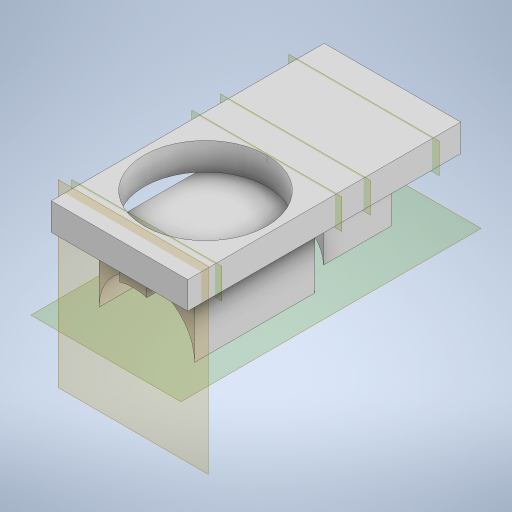
# Autodesk Inventor part: dcmotor_housing_lid
Saved by Autodesk Inventor 2023 (Build 270158000, 158)
## iProperties
Created: 2023-03-20
Part Number: dcmotor_housing_lid
Material: Generic
Document SubType Name: Modeling
Designer: caleb
Density: 1 g/cm^3
Appearance: Default
Author: caleb
Autodesk Inventor part; units mm, degrees
ref_plane "YZ Plane" through (0, 0, 0) normal (1, 0, 0) x (0, 1, 0)
ref_plane "XZ Plane" through (0, 0, 0) normal (0, 1, 0) x (-1, 0, 0)
ref_plane "XY Plane" through (0, 0, 0) normal (0, 0, 1) x (1, 0, 0)
sketch "Sketch1" plane through (0, 0, 0) normal (0, 1, 0) x (-1, 0, 0)
  line L0 (0, 0) -> (50, 0)
  line L1 (50, 0) -> (50, -100)
  line L2 (50, -100) -> (0, -100)
  line L3 (0, -100) -> (0, 0)
  line L4 (25, 0) -> (25, -100)
  line L5 (7.5, -54) -> (7.5, -10)
  line L6 (7.5, -10) -> (42.5, -10)
  line L7 (42.5, -10) -> (42.5, -54)
  line L8 (42.5, -54) -> (7.5, -54)
  line L9 (7.5, -54) -> (42.5, -10) construction
  line L10 (7.5, -10) -> (42.5, -54) construction
  line L11 (7.5, -54) -> (51.5, -54) construction
  line L12 (14.75, -64.45) -> (14.75, -89.55)
  line L13 (14.75, -89.55) -> (35.25, -89.55)
  line L14 (35.25, -89.55) -> (35.25, -64.45)
  line L15 (35.25, -64.45) -> (14.75, -64.45)
  line L16 (14.75, -64.45) -> (35.25, -89.55) construction
  line L17 (14.75, -89.55) -> (35.25, -64.45) construction
  line L18 (14.75, -64.45) -> (39.85, -64.45) construction
  line L19 (25, -10) -> (25, -15)
  line L20 (25, -10) -> (30, -10) construction
  line L21 (20, -20) -> (30, -20)
  line L22 (30, -20) -> (30, -10)
  line L23 (30, -10) -> (20, -10)
  line L24 (20, -10) -> (20, -20)
  line L25 (20, -20) -> (30, -10) construction
  line L26 (30, -20) -> (20, -10) construction
  line L27 (20, -20) -> (30, -20) construction
  line L28 (30, -15) -> (20, -15)
  line L29 (20, -10) -> (30, -10)
  line L30 (30, -10) -> (30, -5)
  line L31 (30, -5) -> (20, -5)
  line L32 (20, -5) -> (20, -10)
  line L33 (25, -54) -> (25, -64.45)
  line L34 (30, -54) -> (30, -64.45)
  line L35 (30, -64.45) -> (20, -64.45)
  line L36 (20, -64.45) -> (20, -54)
  line L37 (20, -54) -> (30, -54)
  line L38 (30, -54) -> (20, -64.45) construction
  line L39 (30, -64.45) -> (20, -54) construction
  circle A0 centre (25, -31.5) radius 22.5
  point P0 (25, -32)
  point P1 (25, -77)
  point P2 (25, -77)
  point P3 (25, -59.225)
  dimension "d36" = 45
  dimension "d0" = 50
  dimension "d1" = 100
  dimension "d2" = 44
  dimension "d3" = 90
  dimension "d4" = 35
  dimension "d5" = 10
  dimension "d6" = 25.1
  dimension "d7" = 90
  dimension "d8" = 20.5
  dimension "d9" = 5
  dimension "d10" = 90
  dimension "d11" = 0
  dimension "d23" = 10
  dimension "d24" = 5
  dimension "d25" = 10
  constraints: 80 end point, 14 midpoint, 14 parallel, 6 horizontal, 6 perpendicular, 5 point on line, 4 equal length, 1 coincident, 1 collinear, 1 vertical, 1 vertical alignment, 2 other
  measures "d0" distance of L1.end L3.start
  measures "d1" distance of L0.end L1.end
  measures "d2" distance of L5.start L6.start
  measures "d3" angle of L11 L5
  measures "d4" distance of L6.start L6.end
  measures "d5" distance between parallel lines of L6 L0
  measures "d6" distance of L15.end L17.start
  measures "d7" angle of L12 L18
  measures "d8" distance of L14.start L17.start
  measures "d9" distance of L19.start L19.end
  measures "d10" angle of L19 L20
  measures "d11" distance between parallel lines of L21 L27
  measures "d23" distance of L31.end L30.end
  measures "d24" distance of L30.end L29.end
  measures "d25" distance of L34.end L35.end
extrude "Extrusion1" add sketch "Sketch1" along normal blind 10
ref_plane "Work Plane1" through (-14.75, 0, -89.55) normal (0, 0, -1) x (-1, 0, 0)
ref_plane "Work Plane2" through (-14.75, 0, -64.45) normal (0, 0, -1) x (-1, 0, 0)
ref_plane "Work Plane3" through (-7.5, 0, -54) normal (0, 0, -1) x (-1, 0, 0)
ref_plane "Work Plane4" through (-7.5, 0, -10) normal (0, 0, -1) x (-1, 0, 0)
sketch "Sketch2" plane through (-14.75, 0, -89.55) normal (0, 0, -1) x (-1, 0, 0)
  line L0 (-14.75, 0) -> (35.25, 0) projected
  line L1 (35.25, 0) -> (35.25, 10) projected
  line L2 (-14.75, 10) -> (35.25, 10) projected
  line L3 (-14.75, 0) -> (-14.75, 10) projected
  line L4 (-14.75, 0) -> (35.25, 0)
  line L5 (35.25, 0) -> (35.25, -50)
  line L6 (35.25, -50) -> (-14.75, -50)
  line L7 (-14.75, -50) -> (-14.75, 0)
  line L8 (0, 0) -> (20.5, 0) projected
  circle A0 centre (10.25, -25) radius 10.25
  dimension "d14" = 50
  dimension "d15" = 50
  dimension "d16" = 20.5
  constraints: 8 end point, 2 parallel, 1 centre point, 1 coincident, 1 horizontal, 1 perpendicular
  measures "d14" distance of L5.end L6.end
  measures "d15" distance of L4.end L5.end
  measures "d16" diameter of A0
sketch "Sketch3" plane through (-7.5, 0, -54) normal (0, 0, -1) x (-1, 0, 0)
  line L0 (42.5, 0) -> (-7.5, 0) projected
  line L1 (-7.5, 0) -> (-7.5, 10) projected
  line L2 (42.5, 10) -> (-7.5, 10) projected
  line L3 (42.5, 0) -> (42.5, 10) projected
  line L4 (-7.5, 0) -> (42.5, 0)
  line L5 (42.5, 0) -> (42.5, -50)
  line L6 (42.5, -50) -> (-7.5, -50)
  line L7 (-7.5, -50) -> (-7.5, 0)
  line L8 (0, 0) -> (35, 0) projected
  circle A0 centre (17.5, -25) radius 17.5
  dimension "d17" = 50
  dimension "d18" = 50
  dimension "d19" = 35
  constraints: 8 end point, 2 parallel, 1 centre point, 1 coincident, 1 horizontal, 1 perpendicular
  measures "d17" distance of L5.end L6.end
  measures "d18" distance of L4.end L5.end
  measures "d19" diameter of A0
sketch "Sketch4" plane through (-14.75, 0, -64.45) normal (0, 0, -1) x (-1, 0, 0)
  line L0 (35.25, 0) -> (-14.75, 0) projected
  line L1 (-14.75, 0) -> (-14.75, 10) projected
  line L2 (35.25, 10) -> (-14.75, 10) projected
  line L3 (35.25, 0) -> (35.25, 10) projected
  line L4 (-14.75, 0) -> (35.25, 0)
  line L5 (35.25, 0) -> (35.25, -50)
  line L6 (35.25, -50) -> (-14.75, -50)
  line L7 (-14.75, -50) -> (-14.75, 0)
  circle A0 centre (10.25, -25) radius 5
  dimension "d20" = 50
  dimension "d21" = 50
  dimension "d22" = 10
  constraints: 8 end point, 2 parallel, 1 centre point, 1 coincident, 1 horizontal, 1 perpendicular
  measures "d20" distance of L5.end L6.end
  measures "d21" distance of L4.end L5.end
  measures "d22" diameter of A0
ref_plane "Work Plane5" through (-25, -25, -89.55) normal (0, -1, 0) x (1, 0, 0)
extrude "Extrusion2" add sketch "Sketch1" against normal up to surface (25 mm away) contours L31 L30 A0 L4 | L4 A0 L32 L31 | A0 L30 L6 L4 | L4 L6 L32 A0 | L13 L12 L15 L4 | L4 L15 L14 L13 | L6 L22 L28 L4 | L4 L28 L24 L6 | L15 L36 L8 L4 | L4 L8 L34 L15 | L28 L22 L21 L4 | L4 L21 L24 L28 | L24 L21 L4 A0 L5 L6 | L6 A0 L7 L4 L21 L22 | L6 L7 A0 | A0 L5 L6 | A0 L7 L8 | L8 L5 A0
extrude "Extrusion3" cut sketch "Sketch2" against normal up to surface (25.1 mm away) contours A0
ref_plane "Work Plane6" through (-30, -25, -5) normal (0, 0, 1) x (1, 0, 0)
extrude "Extrusion4" cut sketch "Sketch4" against normal up to surface (59.45 mm away) contours A0
extrude "Extrusion5" cut sketch "Sketch3" against normal up to surface (49 mm away) contours A0
extrude "Extrusion6" cut sketch "Sketch1" along normal up to surface (10 mm away) contours A0 L30 L6 L4 | L4 L6 L32 A0 | L6 L22 L28 L4 | L4 L28 L24 L6 | A0 L6 L30 | L32 L6 A0 | L28 L22 L21 L4 | L4 L21 L24 L28 | L24 L21 L4 A0 L5 L6 | L6 A0 L7 L4 L21 L22 | A0 L7 | L5 A0
body "Solid1"
